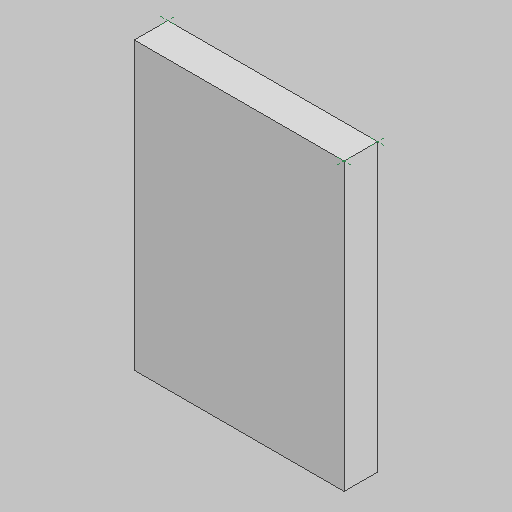
# Autodesk Inventor part: N-Back_into
Saved by Autodesk Inventor 2022 (Build 260153070, 153G)
## iProperties
Created: 2021-11-16
Part Number: N-Back_into
Material: Типовые
Document SubType Name: Modeling
Designer: kalugin_a
Density: 1 g/cm^3
Appearance: По умолчанию
Mass: 3410 g
Surface Area: 2177.8 cm^2
Volume: 3410 cm^3
Author: kalugin_a
Autodesk Inventor part; units mm, degrees
ref_plane "YZ Plane" through (0, 0, 0) normal (1, 0, 0) x (0, 1, 0)
ref_plane "XZ Plane" through (0, 0, 0) normal (0, 1, 0) x (-1, 0, 0)
ref_plane "XY Plane" through (0, 0, 0) normal (0, 0, 1) x (1, 0, 0)
sketch "Эскиз1" plane through (0, 0, 0) normal (0, 0, 1) x (1, 0, 0)
  line L0 (0, 0) -> (250, 0)
  line L1 (250, 0) -> (250, 341)
  line L2 (250, 341) -> (0, 341)
  line L3 (0, 341) -> (0, 0)
  dimension "d0" = 250
  dimension "d1" = 341
  constraints: 8 end point, 2 parallel, 1 horizontal, 1 perpendicular
  measures "d0" distance of L2.end L1.end
  measures "d1" distance of L1.end L0.end
extrude "Выдавливание1" add sketch "Эскиз1" along normal blind 40
sketch "Эскиз2" plane through (0, 341, 0) normal (0, 1, 0) x (1, 0, 0)
  point P0 (0, 0)
  point P1 (250, -40)
  point P2 (250, 0)
